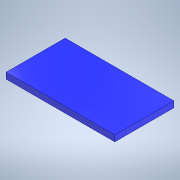
# Autodesk Inventor part: solar_panel
Saved by Autodesk Inventor 2020 (Build 240168000, 168)
## iProperties
Created: 2021-05-30
Part Number: solar_panel
Material: PVC-Piping
Document SubType Name: Modeling
Designer: hasht
Density: 1.4 g/cm^3
Appearance: Blue - Wall Paint - Glossy
Author: hasht
Autodesk Inventor part; units mm, degrees
ref_plane "YZ Plane" through (0, 0, 0) normal (1, 0, 0) x (0, 1, 0)
ref_plane "XZ Plane" through (0, 0, 0) normal (0, 1, 0) x (-1, 0, 0)
ref_plane "XY Plane" through (0, 0, 0) normal (0, 0, 1) x (1, 0, 0)
sketch "Sketch1" plane through (0, 0, 0) normal (0, 1, 0) x (-1, 0, 0)
  line L0 (0, 0) -> (67.818, 0)
  line L1 (67.818, 0) -> (67.818, -36.83)
  line L2 (67.818, -36.83) -> (0, -36.83)
  line L3 (0, -36.83) -> (0, 0)
  dimension "d0" = 67.818
  dimension "d1" = 36.83
  constraints: 8 end point, 2 parallel, 1 horizontal, 1 perpendicular
  measures "d0" distance of L1.end L2.end
  measures "d1" distance of L0.end L1.end
extrude "Extrusion1" add sketch "Sketch1" along normal blind 3.81
body "Solid1"
